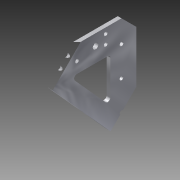
# Autodesk Inventor part: mounting bracket
Saved by Autodesk Inventor 2015 SP1 (Build 190203100, 203)
## iProperties
Created: 2015-01-30
Part Number: mounting bracket
Material: Aluminum 6061
Document SubType Name: Modeling
Designer: Admin
Density: 2.7 g/cm^3
Appearance: Aluminum - Flat
Author: Admin
Autodesk Inventor part; units mm, degrees
ref_plane "YZ Plane" through (0, 0, 0) normal (1, 0, 0) x (0, 1, 0)
ref_plane "XZ Plane" through (0, 0, 0) normal (0, 1, 0) x (-1, 0, 0)
ref_plane "XY Plane" through (0, 0, 0) normal (0, 0, 1) x (1, 0, 0)
sketch "Sketch1" plane through (0, 0, 0) normal (1, 0, 0) x (0, 1, 0)
  line L0 (0, 0) -> (-165.1, 0) construction
  line L1 (-165.1, 0) -> (-165.1, 152.4) construction
  line L2 (-165.1, 152.4) -> (0, 152.4) construction
  line L3 (0, 152.4) -> (0, 0) construction
  line L4 (0, 152.4) -> (-38.1, 152.4)
  line L5 (-165.1, 0) -> (-165.1, 38.1)
  line L6 (-165.1, 38.1) -> (-38.1, 152.4)
  line L7 (0, 152.4) -> (0, 0)
  line L8 (0, 0) -> (-165.1, 0)
  dimension "d0" = 165.1
  dimension "d1" = 152.4
  dimension "d2" = 38.1
  dimension "d3" = 38.1
  constraints: 18 end point, 3 equal length, 2 perpendicular, 2 point on line, 1 horizontal
  measures "d0" distance of L1.end L2.end
  measures "d1" distance of L0.end L1.end
  measures "d2" distance of L2.end L4.end
  measures "d3" distance of L0.end L5.end
extrude "Extrusion1" add sketch "Sketch1" along normal blind 6.35
sketch "Sketch2" plane through (0, 0, 0) normal (-1, 0, 0) x (0, 0, 1)
  line L0 (0, -165.1) -> (0, 0) projected
  line L1 (38.1, -165.1) -> (0, -165.1) projected
  point P0 (25.4, -139.7)
  point P1 (25.4, -88.9)
  point P2 (25.4, -38.1)
  dimension "d6" = 25.4
  dimension "d7" = 25.4
  dimension "d8" = 25.4
  dimension "d9" = 25.4
  dimension "d10" = 50.8
  dimension "d11" = 50.8
  measures "d6" distance from line of L0 point (25.4, -139.7)
  measures "d7" distance from line of L0 point (25.4, -88.9)
  measures "d8" distance from line of L0 point (25.4, -38.1)
  measures "d9" distance from line of L1 point (25.4, -139.7)
  measures "d10" distance of point (25.4, -88.9) point (25.4, -139.7)
  measures "d11" distance of point (25.4, -38.1) point (25.4, -88.9)
hole "Hole1" at (0, -139.7, 25.4) at (0, -88.9, 25.4) at (0, -38.1, 25.4) direction (1, 0, 0) diameter 6.35 end through all
sketch "Sketch3" plane through (0, 0, 0) normal (-1, 0, 0) x (0, 0, 1)
  line L0 (0, -165.1) -> (0, 0) projected
  line L1 (0, 0) -> (25.4, 0)
  line L2 (0, 0) -> (152.4, 0) projected
  line L3 (25.4, 0) -> (0, -25.4)
  line L4 (0, -165.1) -> (0, 0) projected
  line L5 (0, -25.4) -> (0, 0)
  dimension "d19" = 25.4
  dimension "d20" = 45
  constraints: 6 end point, 2 point on line, 1 collinear
  measures "d19" distance of L0.end L1.end
  measures "d20" angle of L1 L3
extrude "Extrusion2" cut sketch "Sketch3" against normal blind 6.35
sketch "Sketch4" plane through (0, 0, 0) normal (-1, 0, 0) x (0, 0, 1)
  line L0 (152.4, 0) -> (152.4, -38.1) projected
  line L1 (25.4, 0) -> (152.4, 0) projected
  point P0 (0, 0)
  point P1 (139.7, -12.7)
  point P2 (127, -25.4)
  point P3 (114.3, -12.7)
  point P4 (101.6, -25.4)
  dimension "d23" = 12.7
  dimension "d24" = 12.7
  dimension "d25" = 25.4
  dimension "d26" = 25.4
  dimension "d27" = 12.7
  dimension "d28" = 38.1
  dimension "d29" = 50.8
  dimension "d30" = 25.4
  measures "d23" distance from line of L0 point (139.7, -12.7)
  measures "d24" distance from line of L1 point (139.7, -12.7)
  measures "d25" distance from line of point (127, -25.4) L0
  measures "d26" distance from line of L1 point (127, -25.4)
  measures "d27" distance from line of L1 point (114.3, -12.7)
  measures "d28" distance from line of point (114.3, -12.7) L0
  measures "d29" distance from line of L0 point (101.6, -25.4)
  measures "d30" distance from line of L1 point (101.6, -25.4)
hole "Hole2" at (0, -12.7, 139.7) at (0, -25.4, 127) at (0, -12.7, 114.3) at (0, -25.4, 101.6) direction (1, 0, 0) diameter 6.35 end through all
sketch "Sketch5" plane through (0, 0, 0) normal (-1, 0, 0) x (0, 0, 1)
  line L0 (0, -165.1) -> (0, -25.4) projected
  line L1 (25.4, 0) -> (152.4, 0) projected
  circle A0 centre (69.85, -19.05) radius 4.7625
  circle A1 centre (52.3875, -25.4) radius 3.175
  circle A2 centre (52.3875, -9.525) radius 3.175
  point P0 (0, 0)
  dimension "d38" = 52.3875
  dimension "d39" = 52.3875
  dimension "d40" = 69.85
  dimension "d41" = 19.05
  dimension "d42" = 9.525
  dimension "d43" = 25.4
  dimension "d44" = 9.525
  dimension "d45" = 6.35
  dimension "d46" = 6.35
  constraints: 3 centre point, 3 coincident
  measures "d38" distance from line of L0 point (52.388, -25.4)
  measures "d39" distance from line of L0 point (52.388, -9.525)
  measures "d40" distance from line of L0 point (69.85, -19.05)
  measures "d41" distance from line of L1 point (69.85, -19.05)
  measures "d42" distance from line of L1 point (52.388, -9.525)
  measures "d43" distance from line of L1 point (52.388, -25.4)
  measures "d44" diameter of A0
  measures "d45" diameter of A1
  measures "d46" diameter of A2
extrude "Extrusion3" cut sketch "Sketch5" against normal blind 6.35
sketch "Sketch6" plane through (0, 0, 0) normal (-1, 0, 0) x (0, 0, 1)
  circle A0 centre (52.3875, -9.525) radius 3.175 projected
  circle A1 centre (52.3875, -25.4) radius 3.175 projected
  circle A2 centre (69.85, -19.05) radius 4.7625 projected
  circle A3 centre (114.3, -12.7) radius 3.175 projected
  circle A4 centre (139.7, -12.7) radius 3.175 projected
  circle A5 centre (127, -25.4) radius 3.175 projected
  circle A6 centre (101.6, -25.4) radius 3.175 projected
  line L0 (25.4, 0) -> (0, -25.4) projected
  line L1 (0, -165.1) -> (0, -25.4) projected
  line L2 (38.1, -165.1) -> (0, -165.1) projected
  line L3 (152.4, -38.1) -> (38.1, -165.1) projected
  line L4 (152.4, 0) -> (152.4, -38.1) projected
  line L5 (25.4, 0) -> (152.4, 0) projected
  circle A7 centre (25.4, -38.1) radius 3.175 projected
  circle A8 centre (25.4, -139.7) radius 3.175 projected
  circle A9 centre (25.4, -88.9) radius 3.175 projected
  line L6 (101.8193, -44.45) -> (49.2125, -44.45)
  line L7 (44.45, -49.2125) -> (44.45, -107.6645)
  line L8 (52.7524, -110.8504) -> (105.3592, -52.3984)
  line L9 (152.4, -38.1) -> (38.1, -38.1) construction
  line L10 (38.1, -38.1) -> (38.1, -165.1) construction
  line L11 (38.1, -165.1) -> (152.4, -165.1) construction
  line L12 (152.4, -165.1) -> (152.4, -38.1) construction
  arc A10 (105.3592, -52.3984) -> (101.8193, -44.45) centre (101.8193, -49.2125) ccw
  arc A11 (49.2125, -44.45) -> (44.45, -49.2125) centre (49.2125, -49.2125) ccw
  arc A12 (44.45, -107.6645) -> (52.7524, -110.8504) centre (49.2125, -107.6645) ccw
  point P0 (0, 0)
  dimension "d49" = 6.35
  dimension "d50" = 6.35
  dimension "d52" = 25.4
  dimension "d53" = 4.7625
  constraints: 14 end point, 6 point on circle, 6 tangent, 3 centre point, 2 equal radius, 2 horizontal, 2 parallel, 2 perpendicular
  measures "d49" distance between parallel lines of L9 L6
  measures "d50" distance between parallel lines of L10 L7
  measures "d52" distance between parallel lines of L3 L8
  measures "d53" radius of A10
extrude "Extrusion4" cut sketch "Sketch6" against normal blind 25.4 contours A10 L8 A12 L7 A11 L6
body "Solid1"
